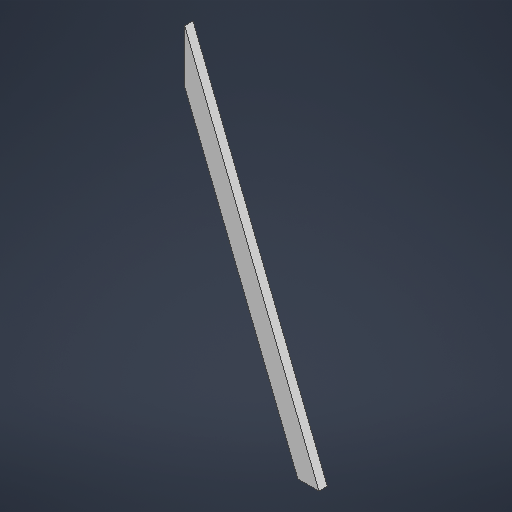
# Autodesk Inventor part: S_2x4x64.622
Saved by Autodesk Inventor 2026 (Build 300175000, 175)
## iProperties
Created: 2025-09-02
Part Number: S_2x4x64.622
Material: Generic
Document SubType Name: Modeling
Designer: trott
Density: 1 g/cm^3
Appearance: Default
Author: trott
Autodesk Inventor part; units mm, degrees
ref_plane "YZ Plane" through (0, 0, 0) normal (1, 0, 0) x (0, 1, 0)
ref_plane "XZ Plane" through (0, 0, 0) normal (0, 1, 0) x (-1, 0, 0)
ref_plane "XY Plane" through (0, 0, 0) normal (0, 0, 1) x (1, 0, 0)
sketch "Sketch1" plane through (0, 0, 0) normal (0, 0, 1) x (1, 0, 0)
  line L0 (0, 0) -> (0, 1524)
  line L1 (0, 0) -> (609.6, 0)
  line L2 (609.6, 0) -> (0, 1524)
  line L3 (609.6, 0) -> (527.0584, -33.0166)
  line L4 (527.0584, -33.0166) -> (0, 1284.6294)
  line L5 (0, 1524) -> (-82.5416, 1490.9834)
  line L6 (0, 1284.6294) -> (-82.5416, 1490.9834)
  point P0 (513.8518, 0)
  dimension "d0" = 1524
  dimension "d1" = 609.6
  dimension "d2" = 88.9
  dimension "d3" = 90
  dimension "d4" = 88.9
  dimension "d5" = 90
  constraints: 14 end point, 1 horizontal, 1 parallel, 1 point on line, 1 vertical
  measures "d0" distance of L0.start L0.end
  measures "d1" distance of L0.start L1.end
  measures "d2" distance of L1.end L3.end
  measures "d3" angle of L2 L3
  measures "d4" distance of L0.end L5.end
  measures "d5" angle of L2 L5
extrude "Extrusion1" add sketch "Sketch1" along normal blind 38.1 contours L0 L2 L1 L4
body "Solid1"
